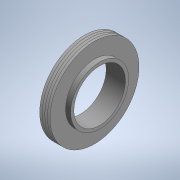
# Autodesk Inventor part: 挡油板2
Saved by Autodesk Inventor 2020 (Build 240168000, 168)
## iProperties
Created: 2021-06-17
Part Number: 挡油板2
Material: 常规
Document SubType Name: Modeling
Designer: dell
Density: 1 g/cm^3
Appearance: 默认
Author: dell
Autodesk Inventor part; units mm, degrees
ref_plane "YZ Plane" through (0, 0, 0) normal (1, 0, 0) x (0, 1, 0)
ref_plane "XZ Plane" through (0, 0, 0) normal (0, 1, 0) x (-1, 0, 0)
ref_plane "XY Plane" through (0, 0, 0) normal (0, 0, 1) x (1, 0, 0)
sketch "草图1" plane through (0, 0, 0) normal (0, 0, 1) x (1, 0, 0)
  line L0 (0, -33.9) -> (0, 45.9) construction
  line L1 (-18, 0) -> (3, 0) construction
  line L2 (0, 22.5) -> (0, -22.5)
  line L3 (0, -22.5) -> (-15, -22.5)
  line L4 (-15, -22.5) -> (-15, 22.5)
  line L5 (-15, 20) -> (0, 20)
  line L6 (0, 20) -> (0, -20)
  line L7 (0, -20) -> (-15, -20)
  line L8 (-15, -20) -> (-15, 20)
  line L9 (-12, 22.5) -> (-12, 34.5)
  line L10 (-12, 34.5) -> (-4, 34.5) construction
  line L11 (-4, 34.5) -> (-4, 22.5)
  line L12 (-12, 34.5) -> (-11, 32.7679)
  line L13 (-11, 32.7679) -> (-10, 34.5)
  line L14 (-10, 34.5) -> (-9, 32.7679)
  line L15 (-9, 32.7679) -> (-8, 34.5)
  line L16 (-8, 34.5) -> (-7, 32.7679)
  line L17 (-7, 32.7679) -> (-6, 34.5)
  line L18 (-6, 34.5) -> (-5, 32.7679)
  line L19 (-5, 32.7679) -> (-4, 34.5)
  line L20 (-15, 22.5) -> (-12, 22.5)
  line L21 (-4, 22.5) -> (0, 22.5)
  point P0 (0, 0)
  point P1 (-8, 34.5)
  dimension "d0" = 40
  dimension "d2" = 15
  dimension "d3" = 3
  dimension "d4" = 8
  dimension "d5" = 34.5
  dimension "d6" = 2
  dimension "d7" = 60
  dimension "d8" = 2
  dimension "d9" = 2
  dimension "d10" = 2
  dimension "d11" = 60
  dimension "d12" = 60
  dimension "d13" = 60
  dimension "d14" = 22.5
  constraints: 40 end point, 6 perpendicular, 5 parallel, 5 point on line, 4 equal length, 3 horizontal, 3 midpoint, 1 collinear, 1 vertical, 1 other
  measures "d0" distance between parallel lines of L7 L5
  measures "d2" distance between parallel lines of L2 L4
  measures "d3" distance between parallel lines of L4 L9
  measures "d4" distance of L9.end L10.end
  measures "d5" distance between parallel lines of L1 L10
  measures "d6" distance of L13.end L9.end
  measures "d7" angle of L10 L12
  measures "d8" distance of L15.end L13.end
  measures "d9" distance of L16.start L17.end
  measures "d10" distance of L10.end L18.start
  measures "d11" angle of L14 L10
  measures "d12" angle of L10 L16
  measures "d13" angle of L10 L18
  measures "d14" distance between parallel lines of L1 L21
revolve "旋转1" add sketch "草图1" angle 360 about axis through (-10, 0, 0) along (1, 0, 0) contours L2 L5 L4 L20 L9 L12 L13 L14 L15 L16 L17 L18 L19 L11 L21
